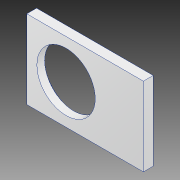
# Autodesk Inventor part: 3102_Biax_Coil_Mounting_Bracket_MPSv2_v1
Saved by Autodesk Inventor 2021 (Build 250183000, 183)
## iProperties
Created: 2020-11-11
Part Number: 3102_Biax_Coil_Mounting_Bracket_MPSv2_v1
Material: Aluminum 6061
Document SubType Name: Modeling
Designer: Admin
Density: 2.7 g/cm^3
Appearance: Aluminum - Flat
Author: Admin
Autodesk Inventor part; units mm, degrees
ref_plane "YZ Plane" through (0, 0, 0) normal (1, 0, 0) x (0, 1, 0)
ref_plane "XZ Plane" through (0, 0, 0) normal (0, 1, 0) x (-1, 0, 0)
ref_plane "XY Plane" through (0, 0, 0) normal (0, 0, 1) x (1, 0, 0)
sketch "Sketch2" plane through (0, 0, 0) normal (0, 0, 1) x (1, 0, 0)
  circle A0 centre (0, 0) radius 18.8587
  circle A1 centre (0, 0) radius 20.6375
  dimension "d0" = 37.7174
  dimension "d1" = 41.275
  constraints: 2 centre point, 2 coincident
  measures "d0" diameter of A0
  measures "d1" diameter of A1
extrude "Extrusion1" add sketch "Sketch2" along normal blind 5
sketch "Sketch3" plane through (0, 0, 0) normal (0, 0, -1) x (-1, 0, 0)
  circle A0 centre (0, 0) radius 20.6375
  circle A1 centre (0, 0) radius 23.1375
  dimension "d4" = 46.275
  constraints: 2 centre point, 2 coincident
  measures "d4" diameter of A1
extrude "Extrusion2" add sketch "Sketch3" along normal blind 1.35 and the other way blind 5
sketch "Sketch10" plane through (0, 0, -1.35) normal (0, 0, -1) x (-1, 0, 0)
  line L0 (-25.4, -25.4) -> (25.4, -25.4)
  line L1 (25.4, -25.4) -> (25.4, 25.4)
  line L2 (25.4, 25.4) -> (-25.4, 25.4)
  line L3 (-25.4, 25.4) -> (-25.4, 0)
  line L4 (-25.4, -25.4) -> (25.4, 25.4) construction
  line L5 (25.4, -25.4) -> (-25.4, 25.4) construction
  line L6 (-25.4, 25.4) -> (-56.5021, 25.4)
  line L7 (-50, -25.4) -> (-25.4, -25.4)
  line L8 (-25.4, 0) -> (-25.4, 25.4)
  line L9 (0, 0) -> (-50, 0)
  line L10 (-50, 0) -> (-50, 25.4)
  line L11 (-50, 0) -> (-50, -25.4)
  circle A0 centre (0, 0) radius 23.1375
  dimension "d46" = 50.8
  dimension "d47" = 50.8
  dimension "d48" = 50
  constraints: 24 end point, 3 horizontal, 3 parallel, 3 point on line, 2 midpoint, 2 perpendicular, 1 centre point, 1 coincident
  measures "d46" distance of L2.end L1.end
  measures "d47" distance of L1.end L0.end
  measures "d48" distance of L9.start L9.end
extrude "Extrusion9" add sketch "Sketch10" against normal blind 6.35
body "Solid1"
